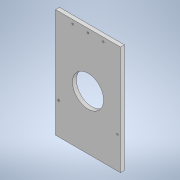
# Autodesk Inventor part: properySideGateGasket
Saved by Autodesk Inventor 2021.2 (Build 252289000, 289)
## iProperties
Created: 2020-11-21
Part Number: properySideGateGasket
Material: Generic
Document SubType Name: Modeling
Designer: robst
Density: 1 g/cm^3
Appearance: Default
Author: robst
Autodesk Inventor part; units mm, degrees
ref_plane "YZ Plane" through (0, 0, 0) normal (1, 0, 0) x (0, 1, 0)
ref_plane "XZ Plane" through (0, 0, 0) normal (0, 1, 0) x (-1, 0, 0)
ref_plane "XY Plane" through (0, 0, 0) normal (0, 0, 1) x (1, 0, 0)
sketch "Sketch2" plane through (0, 0, 0) normal (0, 0, 1) x (1, 0, 0)
  line L0 (-53, -88.9) -> (53, -88.9)
  line L1 (53, -88.9) -> (53, 88.9)
  line L2 (53, 88.9) -> (-53, 88.9)
  line L3 (-53, 88.9) -> (-53, -88.9)
  line L4 (-53, -88.9) -> (53, 88.9) construction
  line L5 (53, -88.9) -> (-53, 88.9) construction
  point P0 (0, 0)
  dimension "d0" = 106
  dimension "d1" = 177.8
  constraints: 12 end point, 2 midpoint, 2 parallel, 1 horizontal, 1 perpendicular
  measures "d0" distance of L2.end L1.end
  measures "d1" distance of L1.end L0.end
extrude "Extrusion1" add sketch "Sketch2" against normal blind 6.35
sketch "Sketch5" plane through (0, 0, 0) normal (0, 0, 1) x (1, 0, 0)
  circle A0 centre (0, 0) radius 25.4
  dimension "d26" = 50.8
  constraints: 1 centre point, 1 coincident
  measures "d26" diameter of A0
extrude "CenterHole" cut sketch "Sketch5" against normal through all
sketch "Sketch6" plane through (0, 0, 0) normal (0, 0, 1) x (1, 0, 0)
  line L0 (-53, 88.9) -> (-53, -88.9) projected
  line L1 (53, -88.9) -> (53, 88.9) projected
  line L2 (-53, -88.9) -> (-53, 88.9) construction
  line L3 (-53, 82.4) -> (53, 82.4) construction
  line L4 (53, 88.9) -> (-53, 88.9) construction
  point P0 (0, 0)
  point P1 (0, 82.4)
  point P2 (123.3454, 23.3667)
  point P3 (-25, 82.4)
  point P4 (25, 82.4)
  dimension "d29" = 6.5
  dimension "d30" = 25
  dimension "d31" = 25
  constraints: 4 point on line, 2 end point, 1 horizontal, 1 midpoint
  measures "d29" distance between parallel lines of L3 L4
  measures "d30" distance of point (-25, 82.4) point (0, 82.4)
  measures "d31" distance of point (25, 82.4) point (0, 82.4)
hole "TopThreeHoles" at (0, 82.4, 0) at (123.3454, 23.3667, 0) at (-25, 82.4, 0) at (25, 82.4, 0) direction (0, 0, -1) diameter 2.6416 end through all thread size "6-32 UNC" class "2B" standard "ANSI Unified Screw Threads"
sketch "Sketch7" plane through (0, 0, 0) normal (0, 0, 1) x (1, 0, 0)
  line L0 (53, -88.9) -> (53, 88.9) projected
  line L1 (-53, 88.9) -> (-53, -88.9) projected
  line L2 (-53, -37.1) -> (53, -37.1) construction
  line L3 (53, 88.9) -> (53, -88.9) projected
  line L4 (53, 88.9) -> (-53, 88.9) construction
  point P0 (0, 0)
  point P1 (-48, -37.1)
  point P2 (48, -37.1)
  dimension "d39" = 126
  dimension "d40" = 5
  dimension "d41" = 5
  constraints: 4 point on line, 2 end point, 1 perpendicular
  measures "d39" distance between parallel lines of L2 L4
  measures "d40" distance from line of point (-48, -37.1) L1
  measures "d41" distance from line of point (48, -37.1) L0
hole "Hole3" at (-48, -37.1, 0) at (48, -37.1, 0) direction (0, 0, -1) diameter 2.6416 end through all thread size "6-32 UNC" class "2B" standard "ANSI Unified Screw Threads"
body "Solid1"
